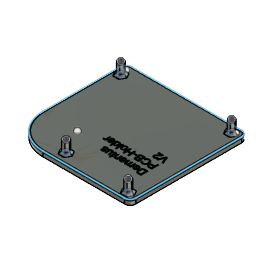
pcb holder_v2 (Autodesk Fusion 360 design; units mm, degrees)
Autodesk Fusion 360 part; units mm, degrees
imported_body "Derived Base Feature1" makes body 1
other "ExternalDerived1"
sketch "Sketch1" plane through (0, 0, 0) normal (0, 0, 1) x (1, 0, 0)
  line L0 (98.5615, -2.034) -> (27.6091, -2.034)
  line L1 (-2.3909, 27.966) -> (-2.3909, 95.1594)
  line L2 (2.6091, 100.1594) -> (98.5615, 100.1594)
  line L3 (103.5615, 95.1594) -> (103.5615, 2.966)
  circle A0 centre (95.9104, 3.9878) radius 1.524
  circle A1 centre (95.9104, 94.0562) radius 1.524
  circle A2 centre (3.9116, 89.535) radius 1.524
  circle A3 centre (39.0144, 6.731) radius 1.524
  line L4 (97.3538, 1.4878) -> (98.7972, 3.9878)
  line L5 (98.7972, 3.9878) -> (97.3538, 6.4878)
  line L6 (97.3538, 6.4878) -> (94.467, 6.4878)
  line L7 (94.467, 6.4878) -> (93.0236, 3.9878)
  line L8 (93.0236, 3.9878) -> (94.467, 1.4878)
  line L9 (94.467, 1.4878) -> (97.3538, 1.4878)
  line L10 (40.4578, 4.231) -> (41.9012, 6.731)
  line L11 (41.9012, 6.731) -> (40.4578, 9.231)
  line L12 (40.4578, 9.231) -> (37.571, 9.231)
  line L13 (37.571, 9.231) -> (36.1276, 6.731)
  line L14 (36.1276, 6.731) -> (37.571, 4.231)
  line L15 (37.571, 4.231) -> (40.4578, 4.231)
  line L16 (5.355, 87.035) -> (6.7984, 89.535)
  line L17 (6.7984, 89.535) -> (5.355, 92.035)
  line L18 (5.355, 92.035) -> (2.4682, 92.035)
  line L19 (2.4682, 92.035) -> (1.0248, 89.535)
  line L20 (1.0248, 89.535) -> (2.4682, 87.035)
  line L21 (2.4682, 87.035) -> (5.355, 87.035)
  line L22 (97.3538, 91.5562) -> (98.7972, 94.0562)
  line L23 (98.7972, 94.0562) -> (97.3538, 96.5562)
  line L24 (97.3538, 96.5562) -> (94.467, 96.5562)
  line L25 (94.467, 96.5562) -> (93.0236, 94.0562)
  line L26 (93.0236, 94.0562) -> (94.467, 91.5562)
  line L27 (94.467, 91.5562) -> (97.3538, 91.5562)
  arc A4 (-2.3909, 27.966) -> (27.6091, -2.034) centre (27.6091, 27.966) ccw
  arc A5 (98.5615, -2.034) -> (103.5615, 2.966) centre (98.5615, 2.966) ccw
  arc A6 (103.5615, 95.1594) -> (98.5615, 100.1594) centre (98.5615, 95.1594) ccw
  arc A7 (2.6091, 100.1594) -> (-2.3909, 95.1594) centre (2.6091, 95.1594) ccw
  point P0 (95.9104, 3.9878)
  point P1 (39.0144, 6.731)
  point P2 (3.9116, 89.535)
  point P3 (95.9104, 94.0562)
  dimension "d1" = 2.5
  dimension "d2" = 2.5
  dimension "d3" = 2.5
  dimension "d4" = 2.5
  dimension "d5" = 30
  dimension "d6" = 5
  constraint horizontal L0
  constraint vertical L1
  constraint horizontal L2
  constraint vertical L3
  constraint coincident P0 A0.centre
  constraint coincident P1 A3.centre
  constraint coincident P2 A2.centre
  constraint coincident P3 A1.centre
  constraint tangent L0 A4
  constraint tangent L1 A4
  constraint tangent L0 A5
  constraint tangent L3 A5
  constraint tangent L2 A6
  constraint tangent L3 A6
  constraint equal A5 A6
  constraint tangent L1 A7
  constraint tangent L2 A7
  constraint equal A5 A7
  measures "d1" distance of P0 L9
  measures "d2" distance of P1 L15
  measures "d3" distance of P2 L21
  measures "d4" distance of P3 L27
  measures "d5" radius of A4
  measures "d6" radius of A5
extrude "Extrude1" add sketch "Sketch1" against normal blind 5 separate body contours L0 L1 L2 L3 A4 A5 A6 A7 | A0 | A1 | A2 | A3 | L4 L5 L6 L7 L8 L9 | L10 L11 L12 L13 L14 L15 | L16 L17 L18 L19 L20 L21 | L22 L23 L24 L25 L26 L27 makes body 2
extrude "Extrude2" add sketch "Sketch1" along normal blind 10 contours A0 | A1 | A2 | A3 | L4 L5 L6 L7 L8 L9 | L10 L11 L12 L13 L14 L15 | L16 L17 L18 L19 L20 L21 | L22 L23 L24 L25 L26 L27 bodies 2
sketch "Sketch2" plane through (0, 0, 10) normal (0, 0, 1) x (-1, 0, 0)
  line L0 (-94.467, -91.5562) -> (-97.3538, -91.5562)
  line L1 (-97.3538, -91.5562) -> (-98.7972, -94.0562)
  line L2 (-98.7972, -94.0562) -> (-97.3538, -96.5562)
  line L3 (-97.3538, -96.5562) -> (-94.467, -96.5562)
  line L4 (-94.467, -96.5562) -> (-93.0236, -94.0562)
  line L5 (-93.0236, -94.0562) -> (-94.467, -91.5562)
  circle A0 centre (-3.9116, -89.535) radius 1.5
  circle A1 centre (-95.9104, -94.0562) radius 1.5
  circle A2 centre (-95.9104, -3.9878) radius 1.5
  circle A3 centre (-39.0144, -6.731) radius 1.5
  circle A4 centre (-95.9104, -3.9878) radius 1
  circle A5 centre (-39.0144, -6.731) radius 1
  circle A6 centre (-3.9116, -89.535) radius 1
  circle A7 centre (-95.9104, -94.0562) radius 1
  point P0 (-95.9104, -94.0562)
  point P1 (-3.9116, -89.535)
  point P2 (-39.0144, -6.731)
  point P3 (-95.9104, -3.9878)
  dimension "d11" = 3
  dimension "d12" = 3
  dimension "d13" = 3
  dimension "d14" = 3
  dimension "d15" = 2
  dimension "d16" = 2
  dimension "d17" = 2
  dimension "d18" = 2
  constraint coincident P1 A0.centre
  constraint coincident P0 A1.centre
  constraint coincident P3 A2.centre
  constraint coincident P2 A3.centre
  measures "d11" diameter of A0
  measures "d12" diameter of A1
  measures "d13" diameter of A2
  measures "d14" diameter of A3
  measures "d15" diameter of A4
  measures "d16" diameter of A5
  measures "d17" diameter of A6
  measures "d18" diameter of A7
extrude "Extrude3" add sketch "Sketch2" along normal blind 1.6 contours A0 | A1 | A2 | A3 bodies 2
extrude "Extrude4" cut sketch "Sketch2" against normal through all contours A4 | A5 | A6 | A7 bodies 2
chamfer "Chamfer1" distance 1 angle 45 8 edges at (-2.3909, 61.5627, 0) (-0.9264, 98.6949, 0) (50.5853, 100.1594, 0) (102.0971, 98.6949, 0) (103.5615, 49.0627, 0) (102.0971, -0.5695, 0) (63.0853, -2.034, 0) (6.3959, 6.7528, 0) on bodies 2
chamfer "Chamfer1" distance 0.5 angle 45 8 edges at (63.0853, -2.034, -5) (6.3959, 6.7528, -5) (-2.3909, 61.5627, -5) (-0.9264, 98.6949, -5) (50.5853, 100.1594, -5) (102.0971, 98.6949, -5) (103.5615, 49.0627, -5) (102.0971, -0.5695, -5) on bodies 2
chamfer "Chamfer1" distance 2 angle 45 24 edges at (39.0144, 4.231, 0) (36.8493, 5.481, 0) (36.8493, 7.981, 0) (39.0144, 9.231, 0) (41.1795, 5.481, 0) (41.1795, 7.981, 0) (95.9104, 6.4878, 0) (93.7453, 5.2378, 0) (98.0755, 5.2378, 0) (95.9104, 1.4878, 0) (98.0755, 2.7378, 0) (93.7453, 2.7378, 0) (95.9104, 91.5562, 0) (93.7453, 92.8062, 0) (93.7453, 95.3062, 0) (95.9104, 96.5562, 0) (98.0755, 92.8062, 0) (98.0755, 95.3062, 0) (6.0767, 90.785, 0) (6.0767, 88.285, 0) (3.9116, 87.035, 0) (1.7465, 88.285, 0) (3.9116, 92.035, 0) (1.7465, 90.785, 0) on bodies 2
sketch "Sketch3" plane through (0, 0, 0) normal (0, 0, 1) x (1, 0, 0)
  line L0 (89.0793, 76.7914) -> (17.8936, 76.7914) construction
  line L1 (17.8936, 76.7914) -> (17.8936, 22.4603) construction
  line L2 (17.8936, 22.4603) -> (89.0793, 22.4603) construction
  line L3 (89.0793, 22.4603) -> (89.0793, 76.7914) construction
  dimension "d25" = 6
  text T0 "Dementus\nPCB-Holder\nV2" font "Arial" height 6 align left top in box 71.1857 x 54.3311 at (89.0793, 76.7914) x (-1, 0) y (0, -1) spacing 1
extrude "Extrude5" cut sketch "Sketch3" against normal blind 0.5 text T0 bodies 2
hidden bodies 1
named bodies: "Płytka"
